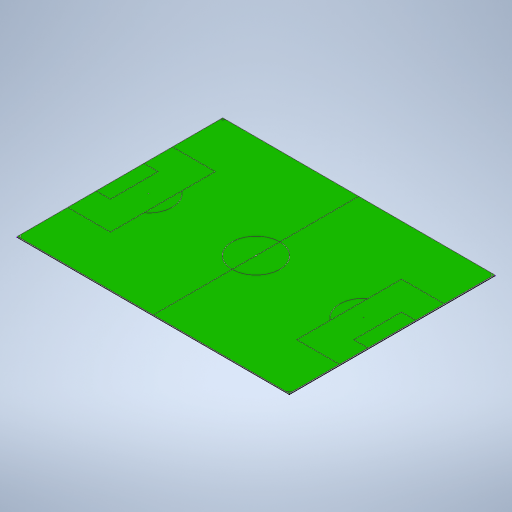
# Autodesk Inventor part: stadium
Saved by Autodesk Inventor 2024.1 (Build 281209000, 209)
## iProperties
Created: 2023-11-12
Part Number: stadium
Material: Generic
Document SubType Name: Modeling
Designer: ASUS
Density: 1 g/cm^3
Appearance: Default
Author: ASUS
Autodesk Inventor part; units mm, degrees
ref_plane "YZ Plane" through (0, 0, 0) normal (1, 0, 0) x (0, 1, 0)
ref_plane "XZ Plane" through (0, 0, 0) normal (0, 1, 0) x (-1, 0, 0)
ref_plane "XY Plane" through (0, 0, 0) normal (0, 0, 1) x (1, 0, 0)
sketch "Sketch2" plane through (0, 0, 0) normal (0, 1, 0) x (-1, 0, 0)
  line L0 (0, 0) -> (52499.9966, 0)
  line L1 (52499.9966, 0) -> (52499.9966, -79350.0064)
  line L2 (52499.9966, -79350.0064) -> (0, -79350.0064)
  line L3 (0, -79350.0064) -> (0, 0)
  line L4 (0, -19525.0054) -> (16500, -19525.0054)
  line L5 (16500, -19525.0054) -> (16500, -59825.001)
  line L6 (16500, -59825.001) -> (0, -59825.001)
  line L7 (0, -30507.1958) -> (5499.9992, -30507.1958)
  line L8 (5499.9992, -30507.1958) -> (5499.9992, -48807.1998)
  line L9 (5499.9992, -48807.1998) -> (0, -48807.1998)
  circle A0 centre (10999.9958, -39675.0032) radius 127
  arc A1 (1000, -79350.0064) -> (0, -78350.0064) centre (0, -79350.0064) ccw
  arc A2 (0, -1000) -> (1000, 0) centre (0, 0) ccw
  arc A3 (16500, -46987.4982) -> (16500, -32362.5082) centre (10999.9958, -39675.0032) ccw
  arc A4 (52499.9966, -30525.0037) -> (52499.9966, -48825.0027) centre (52499.9966, -39675.0032) ccw
  arc A5 (52499.9966, -30398.0037) -> (52499.9966, -48952.0027) centre (52499.9966, -39675.0032) ccw
  arc A6 (52499.9966, -39421.0032) -> (52499.9966, -39929.0032) centre (52499.9966, -39675.0032) ccw
  arc A7 (16576.3388, -47088.9939) -> (16576.3388, -32261.0125) centre (10999.9958, -39675.0032) ccw
  line L10 (0, -59952.001) -> (16627, -59952.001)
  line L11 (16627, -59952.001) -> (16627, -19398.0054)
  line L12 (16627, -19398.0054) -> (0, -19398.0054)
  line L13 (0, -48934.1998) -> (5626.9992, -48934.1998)
  line L14 (5626.9992, -48934.1998) -> (5626.9992, -30380.1958)
  line L15 (5626.9992, -30380.1958) -> (0, -30380.1958)
  arc A8 (0, -1127) -> (1127, 0) centre (0, 0) ccw
  arc A9 (1127, -79350.0064) -> (0, -78223.0064) centre (0, -79350.0064) ccw
  line L16 (127, -127) -> (52436.4966, -127)
  line L17 (52436.4966, -127) -> (52436.4966, -79223.0064)
  line L18 (52436.4966, -79223.0064) -> (127, -79223.0064)
  line L19 (127, -79223.0064) -> (127, -127)
  line L20 (104999.9932, 0) -> (52499.9966, 0)
  line L21 (52499.9966, -79350.0064) -> (104999.9932, -79350.0064)
  line L22 (104999.9932, -79350.0064) -> (104999.9932, 0)
  line L23 (104999.9932, -19525.0054) -> (88499.9932, -19525.0054)
  line L24 (88499.9932, -19525.0054) -> (88499.9932, -59825.001)
  line L25 (88499.9932, -59825.001) -> (104999.9932, -59825.001)
  line L26 (104999.9932, -30507.1958) -> (99499.994, -30507.1958)
  line L27 (99499.994, -30507.1958) -> (99499.994, -48807.1998)
  line L28 (99499.994, -48807.1998) -> (104999.9932, -48807.1998)
  circle A10 centre (93999.9974, -39675.0032) radius 127
  arc A11 (104999.9932, -78350.0064) -> (103999.9932, -79350.0064) centre (104999.9932, -79350.0064) ccw
  arc A12 (103999.9932, 0) -> (104999.9932, -1000) centre (104999.9932, 0) ccw
  arc A13 (88499.9932, -32362.5082) -> (88499.9932, -46987.4982) centre (93999.9974, -39675.0032) ccw
  arc A14 (52499.9966, -48825.0027) -> (52499.9966, -30525.0037) centre (52499.9966, -39675.0032) ccw
  arc A15 (52499.9966, -48952.0027) -> (52499.9966, -30398.0037) centre (52499.9966, -39675.0032) ccw
  arc A16 (52499.9966, -39929.0032) -> (52499.9966, -39421.0032) centre (52499.9966, -39675.0032) ccw
  arc A17 (88423.6544, -32261.0125) -> (88423.6544, -47088.9939) centre (93999.9974, -39675.0032) ccw
  line L29 (104999.9932, -59952.001) -> (88372.9932, -59952.001)
  line L30 (88372.9932, -59952.001) -> (88372.9932, -19398.0054)
  line L31 (88372.9932, -19398.0054) -> (104999.9932, -19398.0054)
  line L32 (104999.9932, -48934.1998) -> (99372.994, -48934.1998)
  line L33 (99372.994, -48934.1998) -> (99372.994, -30380.1958)
  line L34 (99372.994, -30380.1958) -> (104999.9932, -30380.1958)
  arc A18 (103872.9932, 0) -> (104999.9932, -1127) centre (104999.9932, 0) ccw
  arc A19 (104999.9932, -78223.0064) -> (103872.9932, -79350.0064) centre (104999.9932, -79350.0064) ccw
  line L35 (104872.9932, -127) -> (52563.4966, -127)
  line L36 (52563.4966, -127) -> (52563.4966, -79223.0064)
  line L37 (52563.4966, -79223.0064) -> (104872.9932, -79223.0064)
  line L38 (104872.9932, -79223.0064) -> (104872.9932, -127)
  point P0 (52436.4966, -30398.221)
  point P1 (1127, 0)
  point P2 (1119.8214, -127)
  point P3 (52436.4966, -30525.2241)
  point P4 (52436.4966, -48951.7854)
  point P5 (52436.4966, -48824.7823)
  point P6 (52436.4966, -39429.0688)
  point P7 (52436.4966, -39920.9376)
  point P8 (1119.8214, -79223.0064)
  point P9 (127, -78358.1037)
  point P10 (127, -78230.185)
  point P11 (0, -78223.0064)
  point P12 (991.9027, -79223.0064)
  point P13 (127, -59952.001)
  point P14 (127, -991.9027)
  point P15 (991.9027, -127)
  point P16 (127, -1119.8214)
  point P17 (0, -1127)
  point P18 (127, -19398.0054)
  point P19 (127, -19525.0054)
  point P20 (16627, -32459.7795)
  point P21 (127, -30380.1958)
  point P22 (16627, -46890.2269)
  point P23 (16627, -47050.6173)
  point P24 (16627, -32299.3891)
  point P25 (127, -59825.001)
  point P26 (127, -30507.1958)
  point P27 (127, -48807.1998)
  point P28 (127, -48934.1998)
  point P29 (104872.9932, -48934.1998)
  point P30 (104872.9932, -59825.001)
  point P31 (104872.9932, -19525.0054)
  point P32 (104872.9932, -30380.1958)
  point P33 (52563.4966, -30525.2241)
  point P34 (52563.4966, -48824.7823)
  point P35 (52563.4966, -39920.9376)
  point P36 (52563.4966, -39429.0688)
  point P37 (52563.4966, -30398.221)
  point P38 (103880.1718, -127)
  point P39 (104872.9932, -1119.8214)
  point P40 (104872.9932, -19398.0054)
  point P41 (88372.9932, -32299.3891)
  point P42 (88372.9932, -47050.6173)
  point P43 (104872.9932, -59952.001)
  point P44 (104872.9932, -78230.185)
  point P45 (103880.1718, -79223.0064)
  point P46 (52563.4966, -48951.7854)
  point P47 (104872.9932, -991.9027)
  point P48 (104008.0905, -127)
  point P49 (88372.9932, -46890.2269)
  point P50 (88372.9932, -32459.7795)
  point P51 (104008.0905, -79223.0064)
  point P52 (104872.9932, -78358.1037)
  point P53 (104872.9932, -48807.1998)
  point P54 (104872.9932, -30507.1958)
  constraints: 78 end point, 38 symmetric about line, 36 point on circle, 20 centre point, 11 point on line, 8 coincident, 8 parallel, 6 perpendicular, 4 horizontal, 14 other
extrude "Extrusion68" add sketch "Sketch2" along normal blind 254 contours L0 A2 L16 L19 L3 | L0 A8 L16 A2 | A2 L19 A8 L3 | L0 L1 A5 L17 L16 A8 | L16 A8 L19 A2 | A8 L19 L12 L3 | L20 A18 L35 L36 A15 L1 | L12 L19 L4 L3 | A15 L36 A14 L1 | L1 A4 L17 A5 | L20 A12 L35 A18 | L4 L19 L15 L3 | L12 L11 A3 L5 L4 L19 | A14 L36 A16 L1 | L1 A6 L17 A4 | L17 A4 A5 | A15 L36 A14 | L20 L22 A12 L38 L35 | L35 A12 L38 A18 | L15 L19 L7 L3 | A16 L36 L1 | L1 A6 L17 | L17 A4 L1 A5 | A5 L1 L2 A9 L18 L17 | L36 L37 A19 L21 L1 A15 | A15 L1 A14 L36 | L38 A12 L22 A18 | A18 L22 L31 L38 | L7 L19 L9 L3 | L15 L14 L13 L19 L9 L8 L7 | A7 L11 A3 | A16 L36 A14 L1 | L1 A4 L17 A6 | L17 A6 | A16 L36 | L38 L23 L24 A13 L30 L31 | L31 L22 L23 L38 | L9 L19 L13 L3 | A3 L11 L5 | L11 L10 L19 L6 L5 A3 | L18 A1 L19 A9 | A9 L2 A1 L18 | L37 A11 L21 A19 | A19 L38 A11 L37 | L23 L22 L34 L38 | L13 L19 L6 L3 | L19 A1 L3 A9 | A9 L3 L10 L19 | A1 L2 L3 L19 L18 | L38 L29 L22 A19 | A19 L22 A11 L38 | L37 L38 A11 L22 L21 | L30 A13 A17 | L38 L26 L27 L28 L32 L33 L34 | L34 L22 L26 L38 | L6 L19 L10 L3 | L38 L25 L22 L29 | L29 L30 A13 L24 L25 L38 | A13 L24 L30 | L26 L22 L28 L38 | L38 L32 L22 L25 | L28 L22 L32 L38 | A0 | A10
extrude "Extrusion69" add sketch "Sketch2" along normal blind 254 separate body contours A2 L19 L16 | L16 L17 A5 L18 A9 L19 L10 L11 A7 L12 A8 | L36 L35 A18 L38 L31 L30 A17 L29 A19 L37 A15 | L4 L5 L6 L19 L13 L14 L15 | L17 A6 A4 | A14 L36 A16 | L35 L38 A12 | L7 L8 L9 L19 | A3 L11 | L38 L34 L33 L32 L25 L24 L23 | L18 L19 A1 | A11 L38 L37 | L30 A13 | L38 L28 L27 L26
body "Solid12"
body "Solid13"
